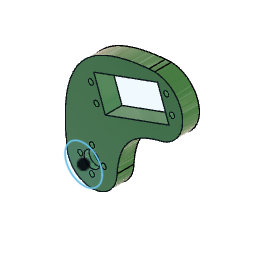
femur v8 (Autodesk Fusion 360 design; units mm, degrees)
Autodesk Fusion 360 part; units mm, degrees
sketch "Sketch1" plane through (0, 0, 0) normal (0, 1, 0) x (1, 0, 0)
  line L0 (0, 0) -> (2.9555, -2.5932)
  spline S0 degree 5 poles (-11.1601, -10.0226) (-9.6312, -16.6468) (-6.2668, -29.3346) (-0.3006, -46.6842) (9.5237, -66.3984) (23.0159, -82.4928) (35.3478, -91.2889) (44.9675, -95.6247) (50.7777, -97.5072) (52.2318, -97.9359) knots 0 0 0 0 0 0 0.1 0.2 0.3 0.4 0.43278 0.43278 0.43278 0.43278 0.43278 0.43278
  line L1 (42.168, -94.9684) -> (62.2956, -100.9035)
  spline S1 degree 5 poles (13.8295, 5.809) (15.3774, 1.0599) (18.5864, -8.2354) (23.7389, -21.57) (31.3341, -38.0483) (42.6284, -55.4164) (54.0114, -65.0989) (64.5325, -68.8015) (72.5693, -69.4349) (76.8436, -69.2924) knots 0 0 0 0 0 0 0.2 0.4 0.6 0.8 1 1 1 1 1 1
  line L2 (65.3591, -69.6752) -> (88.3282, -68.9096)
  arc A0 (14.5735, 3.5514) -> (-11.1601, -10.0226) centre (0, 0) ccw
  line L3 (2.9555, -2.5932) -> (9.43, -11.6651)
  spline S2 degree 2 poles (52.2318, -97.9359) (81.8647, -106.674) (76.8436, -69.2924) knots 0 0 0 4.388663 4.388663 4.388663 weights 1 0.651124 1
  dimension "d1" = 30
  constraint coincident L0.start A0.centre
  constraint midpoint S0.end L1
  constraint midpoint S1.end L2
  constraint coincident S1.start A0
  constraint coincident S1 A0.start
  measures "d1" diameter of A0
extrude "Extrude1" add sketch "Sketch1" along normal blind 10 contours S0 S1 A0 S2
sketch "Sketch2" plane through (0, 0, 0) normal (0, 1, 0) x (1, 0, 0)
  line L0 (67.9285, -91.4423) -> (29.3481, -80.8805)
  line L1 (139.5702, 10.2234) -> (139.4895, 0.2737)
  line L2 (29.3481, -80.8805) -> (34.8993, -82.4001)
  line L3 (29.3481, -80.8805) -> (34.6291, -61.5903)
  line L4 (67.9285, -91.4423) -> (73.2095, -72.1521)
  line L5 (34.6291, -61.5903) -> (73.2095, -72.1521)
  dimension "d7" = 20
  dimension "d8" = 20
  constraint coincident L0 L2.end
  constraint parallel L0 L2
  constraint perpendicular L0 L3
  constraint perpendicular L0 L4
  constraint perpendicular L4 L5
  measures "d7" distance of L0.end L3.end
  measures "d8" distance of L0.start L4.end
extrude "Extrude2" add 1 faces at (8.0926, 10, 6.7359) along direction (0, 1, 0) blind 10
extrude "Extrude3" cut sketch "Sketch2" along normal blind 33
sketch "Sketch3" plane through (0, 0, 0) normal (0, 1, 0) x (1, 0, 0)
  line L0 (29.3481, -80.8805) -> (34.6146, -61.6006)
  line L1 (34.6146, -61.6006) -> (31.9814, -71.2405)
  line L2 (31.9814, -71.2405) -> (33.2989, -66.4173)
  line L3 (33.2989, -66.4173) -> (29.4403, -65.3632)
  circle A0 centre (29.4403, -65.3632) radius 1.5
  line L4 (31.9814, -71.2405) -> (70.5126, -81.7658)
  line L5 (70.5126, -81.7658) -> (71.8302, -76.9425)
  line L6 (71.8302, -76.9425) -> (75.6888, -77.9965)
  circle A1 centre (75.6888, -77.9965) radius 0.9659
  circle A2 centre (26.8052, -75.0098) radius 1.5
  dimension "d13" = 5
  dimension "d14" = 4
  dimension "d15" = 3
  dimension "d16" = 5
  dimension "d17" = 4
  constraint midpoint L0 L1.end
  constraint parallel L1 L2
  constraint perpendicular L0 L3
  constraint coincident L3.end A0.centre
  constraint perpendicular L0 L4
  constraint perpendicular L4 L5
  constraint perpendicular L5 L6
  constraint coincident L6.end A1.centre
  constraint symmetric A0 L4 A2
  measures "d13" distance of L1.end L2.end
  measures "d14" distance of L2.end L3.end
  measures "d15" diameter of A0
  measures "d16" distance of L4.end L5.end
  measures "d17" distance of L5.end L6.end
extrude "Extrude4" cut sketch "Sketch3" along normal blind 30
sketch "Sketch4" plane through (0, 20, 0) normal (0, 1, 0) x (-1, 0, 0)
  circle A0 centre (-26.8052, 75.0098) radius 1.5
  circle A1 centre (-29.4403, 65.3632) radius 1.5
  circle A2 centre (-75.6888, 77.9965) radius 0.9659
  line L0 (-29.3481, 80.8805) -> (-34.6291, 61.5903)
  line L1 (-34.6291, 61.5903) -> (-73.2095, 72.1521)
  line L2 (-73.2095, 72.1521) -> (-67.9285, 91.4423)
  line L3 (-67.9285, 91.4423) -> (-29.3481, 80.8805)
  arc A3 (-13.8295, -5.809) -> (11.1601, 10.0226) centre (0, 0) ccw
  spline S0 degree 5 poles (11.1601, 10.0226) (9.6312, 16.6468) (6.2668, 29.3346) (0.3006, 46.6842) (-9.5237, 66.3984) (-23.0159, 82.4928) (-35.3478, 91.2889) (-44.9675, 95.6247) (-50.7777, 97.5072) (-52.2318, 97.9359) knots 0 0 0 0 0 0 0.1 0.2 0.3 0.4 0.43278 0.43278 0.43278 0.43278 0.43278 0.43278
  spline S1 degree 2 poles (-52.2318, 97.9359) (-81.8647, 106.674) (-76.8436, 69.2924) knots 0 0 0 4.388663 4.388663 4.388663 weights 1 0.651124 1
  spline S2 degree 5 poles (-76.8436, 69.2924) (-72.5693, 69.4349) (-64.5325, 68.8015) (-54.0114, 65.0989) (-42.6284, 55.4164) (-31.5498, 38.3799) (-24.1022, 22.3551) (-19.0799, 9.5054) (-15.9932, 0.7092) (-14.5735, -3.5514) knots -1 -1 -1 -1 -1 -1 -0.8 -0.6 -0.4 -0.2 -0.019093 -0.019093 -0.019093 -0.019093 -0.019093 -0.019093
  spline S3 degree 5 poles (-14.5735, -3.5514) (-14.4237, -4.0011) (-14.2744, -4.4517) (-14.1256, -4.9032) (-13.9773, -5.3557) (-13.8295, -5.809) knots -0.019093 -0.019093 -0.019093 -0.019093 -0.019093 -0.019093 0 0 0 0 0 0
  circle A4 centre (0, 0) radius 10
  line L4 (0, 0) -> (7, 0)
  circle A5 centre (7, 0) radius 1.5
  circle A6 centre (0, 0) radius 2.5
  line L5 (0, 0) -> (0, 0.4217)
  line L6 (0, 0.4217) -> (0, 7.4217)
  circle A7 centre (0, 7.4217) radius 1.5
  circle A8 centre (-7, 0) radius 1.5
  circle A9 centre (0, -7.4217) radius 1.5
  dimension "d20" = 20
  dimension "d21" = 7
  dimension "d22" = 3
  dimension "d23" = 5
  dimension "d24" = 7
  dimension "d25" = 3
  constraint coincident A3.centre A4.centre
  constraint horizontal L4
  constraint coincident L4.end A5.centre
  constraint concentric A4 A6
  constraint perpendicular L4 L5
  constraint perpendicular L4 L6
  constraint coincident L6.end A7.centre
  constraint symmetric A5 L6 A8
  constraint symmetric L4 A7 A9
  measures "d20" diameter of A4
  measures "d21" distance of A3.centre L4.end
  measures "d22" diameter of A5
  measures "d23" diameter of A6
  measures "d24" distance of L5.end L6.end
  measures "d25" diameter of A7
extrude "Extrude5" cut sketch "Sketch4" against normal blind 7 contours A4
extrude "Extrude6" cut 1 faces at (8.0926, 0, 6.7359) along direction (0, 1, 0) blind 5
extrude "Extrude7" cut 5 faces at (6.099, 20, -0.5633) (0.6109, 20, -0.5668) (-0.0399, 20, 6.9563) (-7.9271, 20, -0.1069) (0.4505, 20, -6.8921) along direction (0, -1, 0) blind 15
extrude "Extrude8" cut 1 faces at (-4.9871, 13, -4.8634) along direction (0, -1, 0) blind 3
extrude "Extrude9" cut 1 faces at (23.4358, 20, 55.2689) along direction (0, -1, 0) blind 4
extrude "Extrude10" cut 1 faces at (23.3929, 16, 55.1964) along direction (0, -1, 0) blind 1
sketch "Sketch5" plane through (0, 15, 0) normal (0, 1, 0) x (-1, 0, 0)
  arc A0 (-13.8295, -5.809) -> (11.1601, 10.0226) centre (0, 0) ccw
  spline S0 degree 3 poles (-52.2318, 97.9359) (-44.268, 95.5876) (-37.0019, 91.942) (-23.4784, 81.7603) (-17.6471, 75.3929) (-0.805, 51.4751) (6.5312, 30.0781) (11.1601, 10.0226) knots -11.238033 -11.238033 -11.238033 -11.238033 -8.756038 -8.756038 -6.174817 -6.174817 0 0 0 0
  spline S1 degree 3 poles (-76.8436, 69.2924) (-77.2101, 72.0203) (-77.3151, 74.7982) (-76.8873, 80.2968) (-76.3479, 83.0452) (-74.503, 88.1404) (-73.2252, 90.4991) (-70.0645, 94.2672) (-68.3319, 95.7211) (-64.3535, 97.8655) (-62.2013, 98.5089) (-57.3557, 98.9906) (-54.7434, 98.6766) (-52.2318, 97.9359) knots -4.592063 -4.592063 -4.592063 -4.592063 -3.76958 -3.76958 -2.942064 -2.942064 -2.145152 -2.145152 -1.464178 -1.464178 -0.785567 -0.785567 0 0 0 0
  spline S2 degree 3 poles (-14.5735, -3.5514) (-18.3835, 7.8829) (-25.8996, 28.5625) (-39.794, 50.1793) (-44.0341, 55.3762) (-52.3981, 62.5878) (-56.4294, 65.1248) (-66.0755, 68.7682) (-71.3814, 69.4745) (-76.8436, 69.2924) knots -9.601332 -9.601332 -9.601332 -9.601332 -4.951738 -4.951738 -3.089293 -3.089293 -1.639589 -1.639589 0 0 0 0
  spline S3 degree 3 poles (-13.8295, -5.809) (-13.9525, -5.4318) (-14.076, -5.0548) (-14.324, -4.3022) (-14.4485, -3.9267) (-14.5735, -3.5514) knots -0.237702 -0.237702 -0.237702 -0.237702 -0.118672 -0.118672 0 0 0 0
  line L0 (-29.3481, 80.8805) -> (-34.6291, 61.5903)
  line L1 (-34.6291, 61.5903) -> (-73.2095, 72.1521)
  line L2 (-73.2095, 72.1521) -> (-67.9285, 91.4423)
  line L3 (-67.9285, 91.4423) -> (-29.3481, 80.8805)
  circle A1 centre (-75.6888, 77.9965) radius 0.9659
  circle A2 centre (-29.4403, 65.3632) radius 1.5
  circle A3 centre (-26.8052, 75.0098) radius 1.5
  circle A4 centre (0, 0) radius 10
  spline S4 degree 5 poles (-52.2318, 97.9359) (-52.9415, 98.1339) (-54.3394, 98.5029) (-56.3713, 98.9755) (-58.9501, 99.4436) (-61.9532, 99.7528) (-64.7317, 99.7768) (-67.2811, 99.5017) (-69.5985, 98.9096) (-71.6835, 97.9783) (-73.5395, 96.6833) (-75.1706, 95.0082) (-76.5796, 92.9546) (-77.7664, 90.5514) (-78.7254, 87.8686) (-79.4461, 85.0121) (-79.9155, 82.1048) (-80.12, 79.2734) (-80.0476, 76.6329) (-79.6905, 74.271) (-79.0476, 72.235) (-78.3062, 70.8832) (-77.6239, 70.0268) (-77.113, 69.5256) (-76.8436, 69.2924) knots 0 0 0 0 0 0 0.05 0.1 0.15 0.2 0.25 0.3 0.35 0.4 0.45 0.5 0.55 0.6 0.65 0.7 0.75 0.8 0.85 0.9 0.95 1 1 1 1 1 1
  point P0 (-77, 92)
  point P1 (-69, 99)
  point P2 (-80, 77)
  constraint coincident S0.start S1.end
  constraint coincident S1.start S2.end
extrude "Extrude11" add sketch "Sketch5" against normal up to surface (10 mm away) contours S1 S4 picked at (-78.0117, 78.7262)
sketch "Sketch6" plane through (0, 15, 0) normal (0, 1, 0) x (-1, 0, 0)
  arc A0 (-13.8295, -5.809) -> (11.1601, 10.0226) centre (0, 0) ccw
  spline S0 degree 3 poles (-52.2318, 97.9359) (-44.268, 95.5876) (-37.0019, 91.942) (-23.4784, 81.7603) (-17.6471, 75.3929) (-0.805, 51.4751) (6.5312, 30.0781) (11.1601, 10.0226) knots -11.238033 -11.238033 -11.238033 -11.238033 -8.756038 -8.756038 -6.174817 -6.174817 0 0 0 0
  spline S1 degree 3 poles (-53.2502, 98.2112) (-52.9091, 98.1274) (-52.5695, 98.0355) (-52.2318, 97.9359) knots -0.105633 -0.105633 -0.105633 -0.105633 0 0 0 0
  spline S2 degree 5 poles (-53.2502, 98.2112) (-53.7455, 98.3408) (-54.9249, 98.6363) (-56.7437, 99.0421) (-59.124, 99.4615) (-61.9532, 99.7528) (-64.7317, 99.7768) (-67.2811, 99.5017) (-69.5985, 98.9096) (-71.6835, 97.9783) (-73.5395, 96.6833) (-75.1706, 95.0082) (-76.5796, 92.9546) (-77.7664, 90.5514) (-78.7254, 87.8686) (-79.4461, 85.0121) (-79.9155, 82.1048) (-80.12, 79.2734) (-80.0476, 76.6329) (-79.6905, 74.271) (-79.0476, 72.235) (-78.3062, 70.8832) (-77.6239, 70.0268) (-77.113, 69.5256) (-76.8436, 69.2924) knots 0.014477 0.014477 0.014477 0.014477 0.014477 0.014477 0.05 0.1 0.15 0.2 0.25 0.3 0.35 0.4 0.45 0.5 0.55 0.6 0.65 0.7 0.75 0.8 0.85 0.9 0.95 1 1 1 1 1 1
  spline S3 degree 3 poles (-14.5735, -3.5514) (-18.3835, 7.8829) (-25.8996, 28.5625) (-39.794, 50.1793) (-44.0341, 55.3762) (-52.3981, 62.5878) (-56.4294, 65.1248) (-66.0755, 68.7682) (-71.3814, 69.4745) (-76.8436, 69.2924) knots -9.601332 -9.601332 -9.601332 -9.601332 -4.951738 -4.951738 -3.089293 -3.089293 -1.639589 -1.639589 0 0 0 0
  spline S4 degree 3 poles (-13.8295, -5.809) (-13.9525, -5.4318) (-14.076, -5.0548) (-14.324, -4.3022) (-14.4485, -3.9267) (-14.5735, -3.5514) knots -0.237702 -0.237702 -0.237702 -0.237702 -0.118672 -0.118672 0 0 0 0
  line L0 (-29.3481, 80.8805) -> (-34.6291, 61.5903)
  line L1 (-34.6291, 61.5903) -> (-73.2095, 72.1521)
  line L2 (-73.2095, 72.1521) -> (-67.9285, 91.4423)
  line L3 (-67.9285, 91.4423) -> (-29.3481, 80.8805)
  circle A1 centre (-75.6888, 77.9965) radius 0.9659
  circle A2 centre (-29.4403, 65.3632) radius 1.5
  circle A3 centre (-26.8052, 75.0098) radius 1.5
  circle A4 centre (0, 0) radius 10
  circle A5 centre (-75.6888, 77.9965) radius 1.5
  dimension "d40" = 3
  constraint concentric A1 A5
  measures "d40" diameter of A5
extrude "Extrude12" cut sketch "Sketch6" against normal blind 16 contours A5
sketch "Sketch7" plane through (0, 15, 0) normal (0, 1, 0) x (-1, 0, 0)
  circle A0 centre (-75.6888, 77.9965) radius 1.5
  arc A1 (-13.8295, -5.809) -> (11.1601, 10.0226) centre (0, 0) ccw
  spline S0 degree 3 poles (-52.2318, 97.9359) (-44.268, 95.5876) (-37.0019, 91.942) (-23.4784, 81.7603) (-17.6471, 75.3929) (-0.805, 51.4751) (6.5312, 30.0781) (11.1601, 10.0226) knots -11.238033 -11.238033 -11.238033 -11.238033 -8.756038 -8.756038 -6.174817 -6.174817 0 0 0 0
  spline S1 degree 3 poles (-53.2502, 98.2112) (-52.9091, 98.1274) (-52.5695, 98.0355) (-52.2318, 97.9359) knots -0.105633 -0.105633 -0.105633 -0.105633 0 0 0 0
  spline S2 degree 5 poles (-53.2502, 98.2112) (-53.7455, 98.3408) (-54.9249, 98.6363) (-56.7437, 99.0421) (-59.124, 99.4615) (-61.9532, 99.7528) (-64.7317, 99.7768) (-67.2811, 99.5017) (-69.5985, 98.9096) (-71.6835, 97.9783) (-73.5395, 96.6833) (-75.1706, 95.0082) (-76.5796, 92.9546) (-77.7664, 90.5514) (-78.7254, 87.8686) (-79.4461, 85.0121) (-79.9155, 82.1048) (-80.12, 79.2734) (-80.0476, 76.6329) (-79.6905, 74.271) (-79.0476, 72.235) (-78.3062, 70.8832) (-77.6239, 70.0268) (-77.113, 69.5256) (-76.8436, 69.2924) knots 0.014477 0.014477 0.014477 0.014477 0.014477 0.014477 0.05 0.1 0.15 0.2 0.25 0.3 0.35 0.4 0.45 0.5 0.55 0.6 0.65 0.7 0.75 0.8 0.85 0.9 0.95 1 1 1 1 1 1
  spline S3 degree 3 poles (-14.5735, -3.5514) (-18.3835, 7.8829) (-25.8996, 28.5625) (-39.794, 50.1793) (-44.0341, 55.3762) (-52.3981, 62.5878) (-56.4294, 65.1248) (-66.0755, 68.7682) (-71.3814, 69.4745) (-76.8436, 69.2924) knots -9.601332 -9.601332 -9.601332 -9.601332 -4.951738 -4.951738 -3.089293 -3.089293 -1.639589 -1.639589 0 0 0 0
  spline S4 degree 3 poles (-13.8295, -5.809) (-13.9525, -5.4318) (-14.076, -5.0548) (-14.324, -4.3022) (-14.4485, -3.9267) (-14.5735, -3.5514) knots -0.237702 -0.237702 -0.237702 -0.237702 -0.118672 -0.118672 0 0 0 0
  line L0 (-29.3481, 80.8805) -> (-34.6291, 61.5903)
  line L1 (-34.6291, 61.5903) -> (-73.2095, 72.1521)
  line L2 (-73.2095, 72.1521) -> (-67.9285, 91.4423)
  line L3 (-67.9285, 91.4423) -> (-29.3481, 80.8805)
  circle A2 centre (-29.4403, 65.3632) radius 1.5
  circle A3 centre (-26.8052, 75.0098) radius 1.5
  circle A4 centre (0, 0) radius 10
  line L4 (-29.4403, 65.3632) -> (-26.7968, 75.0195)
  line L5 (-26.7968, 75.0195) -> (-26.8052, 75.0098)
  line L6 (-26.7968, 75.0195) -> (-26.8052, 75.0098)
  line L7 (-75.6234, 78.0951) -> (-72.9799, 87.7513)
  circle A5 centre (-72.9799, 87.7513) radius 1.5
  dimension "d43" = 3
  constraint coincident A2.centre L4.start
  constraint parallel L0 L4
  constraint coincident A3.centre L5.end
  constraint coincident L7.end A5.centre
  measures "d43" diameter of A5
extrude "Extrude13" cut sketch "Sketch7" against normal blind 20 contours A5
sketch "Sketch8" plane through (0, 15, 0) normal (0, 1, 0) x (-1, 0, 0)
  circle A0 centre (-72.9799, 87.7513) radius 1.5
  circle A1 centre (-75.6888, 77.9965) radius 1.5
  arc A2 (-13.8295, -5.809) -> (11.1601, 10.0226) centre (0, 0) ccw
  spline S0 degree 3 poles (-52.2318, 97.9359) (-44.268, 95.5876) (-37.0019, 91.942) (-23.4784, 81.7603) (-17.6471, 75.3929) (-0.805, 51.4751) (6.5312, 30.0781) (11.1601, 10.0226) knots -11.238033 -11.238033 -11.238033 -11.238033 -8.756038 -8.756038 -6.174817 -6.174817 0 0 0 0
  spline S1 degree 3 poles (-53.2502, 98.2112) (-52.9091, 98.1274) (-52.5695, 98.0355) (-52.2318, 97.9359) knots -0.105633 -0.105633 -0.105633 -0.105633 0 0 0 0
  spline S2 degree 5 poles (-53.2502, 98.2112) (-53.7455, 98.3408) (-54.9249, 98.6363) (-56.7437, 99.0421) (-59.124, 99.4615) (-61.9532, 99.7528) (-64.7317, 99.7768) (-67.2811, 99.5017) (-69.5985, 98.9096) (-71.6835, 97.9783) (-73.5395, 96.6833) (-75.1706, 95.0082) (-76.5796, 92.9546) (-77.7664, 90.5514) (-78.7254, 87.8686) (-79.4461, 85.0121) (-79.9155, 82.1048) (-80.12, 79.2734) (-80.0476, 76.6329) (-79.6905, 74.271) (-79.0476, 72.235) (-78.3062, 70.8832) (-77.6239, 70.0268) (-77.113, 69.5256) (-76.8436, 69.2924) knots 0.014477 0.014477 0.014477 0.014477 0.014477 0.014477 0.05 0.1 0.15 0.2 0.25 0.3 0.35 0.4 0.45 0.5 0.55 0.6 0.65 0.7 0.75 0.8 0.85 0.9 0.95 1 1 1 1 1 1
  spline S3 degree 3 poles (-14.5735, -3.5514) (-18.3835, 7.8829) (-25.8996, 28.5625) (-39.794, 50.1793) (-44.0341, 55.3762) (-52.3981, 62.5878) (-56.4294, 65.1248) (-66.0755, 68.7682) (-71.3814, 69.4745) (-76.8436, 69.2924) knots -9.601332 -9.601332 -9.601332 -9.601332 -4.951738 -4.951738 -3.089293 -3.089293 -1.639589 -1.639589 0 0 0 0
  spline S4 degree 3 poles (-13.8295, -5.809) (-13.9525, -5.4318) (-14.076, -5.0548) (-14.324, -4.3022) (-14.4485, -3.9267) (-14.5735, -3.5514) knots -0.237702 -0.237702 -0.237702 -0.237702 -0.118672 -0.118672 0 0 0 0
  line L0 (-29.3481, 80.8805) -> (-34.6291, 61.5903)
  line L1 (-34.6291, 61.5903) -> (-73.2095, 72.1521)
  line L2 (-73.2095, 72.1521) -> (-67.9285, 91.4423)
  line L3 (-67.9285, 91.4423) -> (-29.3481, 80.8805)
  circle A3 centre (-29.4403, 65.3632) radius 1.5
  circle A4 centre (-26.8052, 75.0098) radius 1.5
  circle A5 centre (0, 0) radius 10
  circle A6 centre (0, 0) radius 11
  dimension "d46" = 22
  constraint concentric A2 A6
  measures "d46" diameter of A6
extrude "Extrude14" cut sketch "Sketch8" against normal blind 5 contours A6
sketch "Sketch9" plane through (0, 10, 0) normal (0, 1, 0) x (-1, 0, 0)
  circle A0 centre (0, 0) radius 11
  circle A1 centre (0, 0) radius 2.5
  circle A2 centre (0, 7.4217) radius 1.5
  circle A3 centre (7, 0) radius 1.5
  circle A4 centre (-7, 0) radius 1.5
  circle A5 centre (0, -7.4217) radius 1.5
  circle A6 centre (0, 0) radius 4
  dimension "d49" = 8
  constraint concentric A0 A6
  measures "d49" diameter of A6
extrude "Extrude15" cut sketch "Sketch9" against normal blind 10 contours A6
sketch "Sketch10" plane through (0, 10, 0) normal (0, 1, 0) x (-1, 0, 0)
  circle A0 centre (0, 0) radius 4
  circle A1 centre (0, 0) radius 11
  circle A2 centre (0, 7.4217) radius 1.5
  circle A3 centre (7, 0) radius 1.5
  circle A4 centre (-7, 0) radius 1.5
  circle A5 centre (0, -7.4217) radius 1.5
  circle A6 centre (7, 0) radius 2
  circle A7 centre (7, 0) radius 2
  circle A8 centre (0, 7.4217) radius 2
  circle A9 centre (-7, 0) radius 2
  circle A10 centre (0, -7.5) radius 2
  point P0 (7, 0)
  dimension "d52" = 4
  dimension "d53" = 4
  dimension "d54" = 4
  dimension "d55" = 4
  dimension "d56" = 4
  constraint concentric A3 A6
  constraint concentric A2 A8
  constraint concentric A4 A9
  measures "d52" diameter of A6
  measures "d53" diameter of A7
  measures "d54" diameter of A8
  measures "d55" diameter of A9
  measures "d56" diameter of A10
extrude "Extrude16" cut sketch "Sketch10" against normal blind 6 contours A6 A7 | A8 | A9 | A10
sketch "Sketch11" plane through (0, 15, 0) normal (0, 1, 0) x (-1, 0, 0)
  circle A0 centre (0, 0) radius 11
  circle A1 centre (-72.9799, 87.7513) radius 1.5
  circle A2 centre (-75.6888, 77.9965) radius 1.5
  arc A3 (-13.8295, -5.809) -> (11.1601, 10.0226) centre (0, 0) ccw
  spline S0 degree 3 poles (-52.2318, 97.9359) (-44.268, 95.5876) (-37.0019, 91.942) (-23.4784, 81.7603) (-17.6471, 75.3929) (-0.805, 51.4751) (6.5312, 30.0781) (11.1601, 10.0226) knots -11.238033 -11.238033 -11.238033 -11.238033 -8.756038 -8.756038 -6.174817 -6.174817 0 0 0 0
  spline S1 degree 3 poles (-53.2502, 98.2112) (-52.9091, 98.1274) (-52.5695, 98.0355) (-52.2318, 97.9359) knots -0.105633 -0.105633 -0.105633 -0.105633 0 0 0 0
  spline S2 degree 5 poles (-53.2502, 98.2112) (-53.7455, 98.3408) (-54.9249, 98.6363) (-56.7437, 99.0421) (-59.124, 99.4615) (-61.9532, 99.7528) (-64.7317, 99.7768) (-67.2811, 99.5017) (-69.5985, 98.9096) (-71.6835, 97.9783) (-73.5395, 96.6833) (-75.1706, 95.0082) (-76.5796, 92.9546) (-77.7664, 90.5514) (-78.7254, 87.8686) (-79.4461, 85.0121) (-79.9155, 82.1048) (-80.12, 79.2734) (-80.0476, 76.6329) (-79.6905, 74.271) (-79.0476, 72.235) (-78.3062, 70.8832) (-77.6239, 70.0268) (-77.113, 69.5256) (-76.8436, 69.2924) knots 0.014477 0.014477 0.014477 0.014477 0.014477 0.014477 0.05 0.1 0.15 0.2 0.25 0.3 0.35 0.4 0.45 0.5 0.55 0.6 0.65 0.7 0.75 0.8 0.85 0.9 0.95 1 1 1 1 1 1
  spline S3 degree 3 poles (-14.5735, -3.5514) (-18.3835, 7.8829) (-25.8996, 28.5625) (-39.794, 50.1793) (-44.0341, 55.3762) (-52.3981, 62.5878) (-56.4294, 65.1248) (-66.0755, 68.7682) (-71.3814, 69.4745) (-76.8436, 69.2924) knots -9.601332 -9.601332 -9.601332 -9.601332 -4.951738 -4.951738 -3.089293 -3.089293 -1.639589 -1.639589 0 0 0 0
  spline S4 degree 3 poles (-13.8295, -5.809) (-13.9525, -5.4318) (-14.076, -5.0548) (-14.324, -4.3022) (-14.4485, -3.9267) (-14.5735, -3.5514) knots -0.237702 -0.237702 -0.237702 -0.237702 -0.118672 -0.118672 0 0 0 0
  line L0 (-29.3481, 80.8805) -> (-34.6291, 61.5903)
  line L1 (-34.6291, 61.5903) -> (-73.2095, 72.1521)
  line L2 (-73.2095, 72.1521) -> (-67.9285, 91.4423)
  line L3 (-67.9285, 91.4423) -> (-29.3481, 80.8805)
  circle A4 centre (-29.4403, 65.3632) radius 1.5
  circle A5 centre (-26.8052, 75.0098) radius 1.5
extrude "Extrude17" cut sketch "Sketch11" against normal blind 25
sketch "Sketch12" plane through (0, 10, 0) normal (0, 1, 0) x (-1, 0, 0)
  circle A0 centre (7, 0) radius 2
  circle A1 centre (0, -7.5) radius 2
  circle A2 centre (-7, 0) radius 2
  circle A3 centre (0, 7.4217) radius 2
  circle A4 centre (0, 0) radius 4
  circle A5 centre (0, 0) radius 11
  circle A6 centre (0, 0) radius 15
  spline S0 degree 5 poles (-15, 0) (-15.06, 0.9359) (-15.2173, 2.7776) (-15.5654, 5.4503) (-16.2574, 8.8308) (-17.528, 12.7308) (-19.2401, 16.2761) (-21.4296, 19.4382) (-24.1154, 22.2017) (-27.2773, 24.5828) (-30.8792, 26.6107) (-34.0836, 27.9737) (-36.6569, 28.8593) (-38.4469, 29.39) (-39.3605, 29.6405) knots 0 0 0 0 0 0 0.1 0.2 0.3 0.4 0.5 0.6 0.7 0.8 0.9 1 1 1 1 1 1
  spline S1 degree 5 poles (-37.4563, 64.0414) (-35.0557, 63.9062) (-30.3729, 63.5355) (-23.7037, 62.6785) (-15.5331, 60.9241) (-6.6041, 57.6424) (0.9269, 53.1756) (6.9476, 47.4285) (11.3995, 40.3515) (14.3483, 32.0003) (15.9089, 22.4723) (16.1387, 13.9864) (15.7746, 7.1672) (15.2973, 2.4222) (15, 0) knots 0 0 0 0 0 0 0.1 0.2 0.3 0.4 0.5 0.6 0.7 0.8 0.9 1 1 1 1 1 1
  arc A7 (-33.9038, 63.793) -> (-39.3605, 29.6405) centre (-36.8798, 46.7563) ccw
  line L0 (-45.9908, 40.7308) -> (-39.1641, 59.5297)
  line L1 (-39.1641, 59.5297) -> (-1.0965, 45.7056)
  line L2 (-1.0965, 45.7056) -> (-7.9232, 26.9067)
  line L3 (-7.9232, 26.9067) -> (-45.9908, 40.7308)
  circle A8 centre (-44.3956, 56.11) radius 1.5
  circle A9 centre (0.7216, 39.7258) radius 1.5
  circle A10 centre (-47.8089, 46.7106) radius 1.5
  circle A11 centre (-2.6917, 30.3264) radius 1.5
  point P0 (-21.5164, 19.2938)
  point P1 (6.4089, 47.2762)
  dimension "d63" = 30
  dimension "d64" = 20
  dimension "d65" = 40.5
  dimension "d66" = 20
  dimension "d73" = 3
  dimension "d74" = 3
  constraint concentric A4 A6
  constraint coincident A6 S0.start
  constraint coincident S1.start A7
  constraint coincident A6 S1.end
  constraint coincident S1 A7.start
  constraint perpendicular L0 L1
  constraint perpendicular L1 L2
  measures "d63" diameter of A6
  measures "d64" distance of L0.start L0.end
  measures "d65" distance of L0.end L1.end
  measures "d66" distance of L1.end L2.end
  measures "d73" diameter of A8
  measures "d74" diameter of A9
extrude "Extrude18" add sketch "Sketch12" against normal blind 5 contours A6 | A6 S0 S1 A7
sketch "Sketch13" plane through (0, 5, 0) normal (0, -1, 0) x (1, 0, 0)
  arc A0 (-15, 0) -> (15, 0) centre (0, 0) ccw
  spline S0 degree 5 poles (15, 0) (15.06, 0.9359) (15.2173, 2.7776) (15.5654, 5.4503) (16.2574, 8.8308) (17.528, 12.7308) (19.2401, 16.2761) (21.4296, 19.4382) (24.1154, 22.2017) (27.2773, 24.5828) (30.8792, 26.6107) (34.0836, 27.9737) (36.6569, 28.8593) (38.4469, 29.39) (39.3605, 29.6405) knots 0 0 0 0 0 0 0.1 0.2 0.3 0.4 0.5 0.6 0.7 0.8 0.9 1 1 1 1 1 1
  arc A1 (39.3605, 29.6405) -> (37.4563, 64.0414) centre (36.8798, 46.7563) ccw
  spline S1 degree 5 poles (37.4563, 64.0414) (36.7351, 64.0008) (36.0193, 63.9556) (35.3087, 63.9059) (34.6036, 63.8517) (33.9038, 63.793) knots 0 0 0 0 0 0 0.030042 0.030042 0.030042 0.030042 0.030042 0.030042
  spline S2 degree 5 poles (33.9038, 63.793) (32.2742, 63.6562) (28.3856, 63.2642) (22.4822, 62.4101) (14.9966, 60.7269) (6.6041, 57.6424) (-0.9269, 53.1756) (-6.9476, 47.4285) (-11.3995, 40.3515) (-14.3483, 32.0003) (-15.9089, 22.4723) (-16.1387, 13.9864) (-15.7746, 7.1672) (-15.2973, 2.4222) (-15, 0) knots 0.030042 0.030042 0.030042 0.030042 0.030042 0.030042 0.1 0.2 0.3 0.4 0.5 0.6 0.7 0.8 0.9 1 1 1 1 1 1
  circle A2 centre (44.3956, 56.11) radius 1.5
  line L0 (7.9232, 26.9067) -> (1.0965, 45.7056)
  line L1 (1.0965, 45.7056) -> (39.1641, 59.5297)
  line L2 (39.1641, 59.5297) -> (45.9908, 40.7308)
  line L3 (45.9908, 40.7308) -> (7.9232, 26.9067)
  circle A3 centre (47.8089, 46.7106) radius 1.5
  circle A4 centre (-0.7216, 39.7258) radius 1.5
  circle A5 centre (2.6917, 30.3264) radius 1.5
  circle A6 centre (-7, 0) radius 2
  circle A7 centre (0, -7.5) radius 2
  circle A8 centre (7, 0) radius 2
  circle A9 centre (0, 7.4217) radius 2
  circle A10 centre (0, 0) radius 4
extrude "Extrude19" add 1 faces at (-4.7388, 10, 20.9441) along direction (0, 1, 0) blind 5
sketch "Sketch14" plane through (0, 15, 0) normal (0, 1, 0) x (-1, 0, 0)
  arc A0 (-15, 0) -> (15, 0) centre (0, 0) ccw
  spline S0 degree 5 poles (15, 0) (15.2973, 2.4222) (15.7746, 7.1672) (16.1387, 13.9864) (15.9089, 22.4723) (14.3483, 32.0003) (11.3995, 40.3515) (6.9476, 47.4285) (0.9269, 53.1756) (-6.6041, 57.6424) (-14.9966, 60.7269) (-22.4822, 62.4101) (-28.3856, 63.2642) (-32.2742, 63.6562) (-33.9038, 63.793) knots -1 -1 -1 -1 -1 -1 -0.9 -0.8 -0.7 -0.6 -0.5 -0.4 -0.3 -0.2 -0.1 -0.030042 -0.030042 -0.030042 -0.030042 -0.030042 -0.030042
  spline S1 degree 5 poles (-33.9038, 63.793) (-34.6036, 63.8517) (-35.3087, 63.9059) (-36.0193, 63.9556) (-36.7351, 64.0008) (-37.4563, 64.0414) knots -0.030042 -0.030042 -0.030042 -0.030042 -0.030042 -0.030042 0 0 0 0 0 0
  arc A1 (-37.4563, 64.0414) -> (-39.3605, 29.6405) centre (-36.8798, 46.7563) ccw
  spline S2 degree 5 poles (-39.3605, 29.6405) (-38.4469, 29.39) (-36.6569, 28.8593) (-34.0836, 27.9737) (-30.8792, 26.6107) (-27.2773, 24.5828) (-24.1154, 22.2017) (-21.4296, 19.4382) (-19.2401, 16.2761) (-17.528, 12.7308) (-16.2574, 8.8308) (-15.5654, 5.4503) (-15.2173, 2.7776) (-15.06, 0.9359) (-15, 0) knots -1 -1 -1 -1 -1 -1 -0.9 -0.8 -0.7 -0.6 -0.5 -0.4 -0.3 -0.2 -0.1 0 0 0 0 0 0
  circle A2 centre (-44.3956, 56.11) radius 1.5
  line L0 (-1.0965, 45.7056) -> (-7.9232, 26.9067)
  line L1 (-7.9232, 26.9067) -> (-45.9908, 40.7308)
  line L2 (-45.9908, 40.7308) -> (-39.1641, 59.5297)
  line L3 (-39.1641, 59.5297) -> (-1.0965, 45.7056)
  circle A3 centre (-47.8089, 46.7106) radius 1.5
  circle A4 centre (0.7216, 39.7258) radius 1.5
  circle A5 centre (-2.6917, 30.3264) radius 1.5
  circle A6 centre (7, 0) radius 2
  circle A7 centre (0, -7.5) radius 2
  circle A8 centre (-7, 0) radius 2
  circle A9 centre (0, 7.4217) radius 2
  circle A10 centre (0, 0) radius 4
  circle A11 centre (0, 0) radius 11
  dimension "d80" = 22
  constraint concentric A0 A11
  measures "d80" diameter of A11
extrude "Extrude20" cut sketch "Sketch14" against normal blind 5 contours A11
extrude "Extrude21" cut 1 faces at (4.3898, 10, 5.63) along direction (0, -1, 0) blind 2
sketch "Sketch15" plane through (0, 5, 0) normal (0, -1, 0) x (1, 0, 0)
  circle A0 centre (0, 0) radius 4.75
  dimension "d85" = 9.5
  constraint coincident A0.centre origin
  measures "d85" diameter of A0
extrude "Extrude22" cut sketch "Sketch15" against normal blind 11
sketch "Sketch16" plane through (0, 8, 0) normal (0, 1, 0) x (-1, 0, 0)
  circle A0 centre (0, 0) radius 4.75
  circle A1 centre (7, 0) radius 2
  circle A2 centre (0, -7.5) radius 2
  circle A3 centre (-7, 0) radius 2
  circle A4 centre (0, 7.4217) radius 2
  circle A5 centre (0, 0) radius 11
  circle A6 centre (0, 7.4217) radius 1.5
  circle A7 centre (0, 7.4217) radius 2
  circle A8 centre (-7, 0) radius 2
  circle A9 centre (-7, 0) radius 1.5
  circle A10 centre (7, 0) radius 1.5
  circle A11 centre (7, 0) radius 2
  circle A12 centre (0, -7.5) radius 2
  circle A13 centre (0, -7.5) radius 1.5
  dimension "d88" = 3
  dimension "d89" = 3
  dimension "d90" = 3
  dimension "d91" = 3
  constraint concentric A4 A6
  constraint concentric A4 A7
  constraint concentric A3 A8
  constraint concentric A8 A9
  constraint concentric A1 A10
  constraint concentric A1 A11
  constraint concentric A2 A12
  constraint concentric A2 A13
  measures "d88" diameter of A6
  measures "d89" diameter of A9
  measures "d90" diameter of A10
  measures "d91" diameter of A13
extrude "Extrude23" add sketch "Sketch16" against normal blind 3 contours A1 A11 | A2 A12 | A3 A8 | A4 A7
sketch "Sketch17" plane through (0, 0, 0) normal (0, 1, 0) x (1, 0, 0)
  circle A0 centre (0, 0) radius 11.0804
  constraint coincident A0.centre origin
